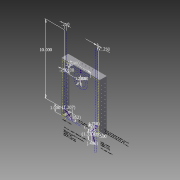
# Autodesk Inventor part: Bay Door Prototype Mk1
Saved by Autodesk Inventor 2015 (Build 190159000, 159)
## iProperties
Created: 2016-11-23
Part Number: Bay Door Prototype Mk1
Material: Generic
Document SubType Name: Modeling
Designer: Markus
Density: 1 g/cm^3
Appearance: Default
Author: Markus
Autodesk Inventor part; units mm, degrees
ref_plane "YZ Plane" through (0, 0, 0) normal (1, 0, 0) x (0, 1, 0)
ref_plane "XZ Plane" through (0, 0, 0) normal (0, 1, 0) x (-1, 0, 0)
ref_plane "XY Plane" through (0, 0, 0) normal (0, 0, 1) x (1, 0, 0)
sketch "Sketch1" plane through (0, 0, 0) normal (0, 0, 1) x (1, 0, 0)
  line L0 (0, 0) -> (142.24, 0)
  line L1 (142.24, 0) -> (142.24, 184.15)
  line L2 (142.24, 184.15) -> (0, 184.15)
  line L3 (0, 184.15) -> (0, 0)
  line L4 (4.3434, 179.8066) -> (137.8966, 179.8066)
  line L5 (137.8966, 179.8066) -> (137.8966, 4.3434)
  line L6 (137.8966, 4.3434) -> (4.3434, 4.3434)
  line L7 (4.3434, 4.3434) -> (4.3434, 179.8066)
  dimension "d0" = 184.15
  dimension "d1" = 142.24
  dimension "d2" = 4.3434
  constraints: 16 end point, 4 parallel, 2 perpendicular, 1 horizontal, 3 other
  measures "d0" distance of L2.end L0.start
  measures "d1" distance of L1.end L2.end
  measures "d2" distance between parallel lines of L2 L4
extrude "Extrusion1" add sketch "Sketch1" along normal blind 25.4
sketch "Sketch2" plane through (0, 0, 25.4) normal (0, 0, 1) x (1, 0, 0)
  line L0 (4.3434, 4.3434) -> (137.8966, 4.3434) projected
  line L1 (14.2875, 4.3434) -> (127.9525, 4.3434)
  line L2 (127.9525, 4.3434) -> (127.9525, 0)
  line L3 (127.9525, 0) -> (14.2875, 0)
  line L4 (14.2875, 0) -> (14.2875, 4.3434)
  line L5 (0, 184.15) -> (0, 0) projected
  line L6 (142.24, 0) -> (142.24, 184.15) projected
  dimension "d5" = 14.2875
  dimension "d6" = 14.2875
  constraints: 8 end point, 2 parallel, 1 horizontal, 1 horizontal alignment, 1 perpendicular, 1 point on line
  measures "d5" distance between parallel lines of L5 L4
  measures "d6" distance between parallel lines of L6 L2
extrude "Extrusion2" cut sketch "Sketch2" against normal up to surface (25.4 mm away)
sketch "Sketch3" plane through (0, 0, 25.4) normal (0, 0, 1) x (1, 0, 0)
  line L0 (10.6934, 279.4) -> (17.0434, 279.4) construction
  line L1 (17.0434, 279.4) -> (17.0434, 25.4) construction
  line L2 (17.0434, 25.4) -> (10.6934, 25.4) construction
  line L3 (10.6934, 25.4) -> (10.6934, 279.4) construction
  line L4 (125.1966, 279.4) -> (131.5466, 279.4) construction
  line L5 (131.5466, 279.4) -> (131.5466, 25.4) construction
  line L6 (131.5466, 25.4) -> (125.1966, 25.4) construction
  line L7 (125.1966, 25.4) -> (125.1966, 279.4) construction
  line L8 (14.2875, 4.3434) -> (71.12, 4.3434) construction
  line L9 (71.12, 4.3434) -> (71.12, 0) construction
  line L10 (71.12, 0) -> (14.2875, 0) construction
  line L11 (14.2875, 0) -> (14.2875, 4.3434) construction
  line L12 (4.3434, 179.8066) -> (137.8966, 179.8066) construction
  line L13 (4.3434, 4.3434) -> (4.3434, 179.8066) construction
  line L14 (0, 0) -> (14.2875, 0) construction
  line L15 (137.8966, 179.8066) -> (137.8966, 4.3434) construction
  line L16 (127.9525, 0) -> (123.6091, 0) construction
  line L17 (123.6091, 0) -> (123.6091, -56.8325) construction
  line L18 (123.6091, -56.8325) -> (127.9525, -56.8325) construction
  line L19 (127.9525, -56.8325) -> (127.9525, 0) construction
  line L20 (137.8966, 4.3434) -> (112.4966, 4.3434) construction
  arc A0 (111.9446, 7.4193) -> (112.4966, 4.3434) centre (112.4966, 5.9309) ccw construction
  line L21 (111.9446, 7.4193) -> (137.8966, 17.0434) construction
  line L22 (137.8966, 4.3434) -> (137.8966, 179.8066) construction
  line L23 (159.3941, 36.0216) -> (266.702, 36.0216) construction
  line L24 (266.702, 36.0216) -> (266.702, 6.9446) construction
  line L25 (266.702, 6.9446) -> (159.3941, 6.9446) construction
  line L26 (159.3941, 6.9446) -> (159.3941, 36.0216) construction
  circle A1 centre (13.8684, 28.575) radius 3.175 construction
  circle A2 centre (128.3716, 28.575) radius 3.175 construction
  line L27 (42.7037, 4.3434) -> (12.0379, 25.9808)
  line L28 (111.3731, 7.0524) -> (130.6186, 26.3319)
  line L29 (111.0091, 5.3763) -> (123.6091, -28.4162)
  line L30 (63.5032, 17.7448) -> (103.5407, 17.7448) construction
  line L31 (103.5407, 17.7448) -> (103.5407, 7.0443) construction
  line L32 (103.5407, 7.0443) -> (63.5032, 7.0443) construction
  line L33 (63.5032, 7.0443) -> (63.5032, 17.7448) construction
  line L34 (144.8974, -10.3874) -> (251.178, -10.3874) construction
  line L35 (251.178, -10.3874) -> (251.178, -62.6009) construction
  line L36 (251.178, -62.6009) -> (144.8974, -62.6009) construction
  line L37 (144.8974, -62.6009) -> (144.8974, -10.3874) construction
  arc A3 (111.3731, 7.0524) -> (111.0091, 5.3763) centre (112.4966, 5.9309) ccw
  line L38 (3.9911, -9.0202) -> (42.7037, -9.0202) construction
  line L39 (42.7037, -9.0202) -> (42.7037, -18.258) construction
  line L40 (42.7037, -18.258) -> (3.9911, -18.258) construction
  line L41 (3.9911, -18.258) -> (3.9911, -9.0202) construction
  line L42 (8.6414, -30.8758) -> (98.6277, -30.8758) construction
  line L43 (98.6277, -30.8758) -> (98.6277, -107.8338) construction
  line L44 (98.6277, -107.8338) -> (8.6414, -107.8338) construction
  line L45 (8.6414, -107.8338) -> (8.6414, -30.8758) construction
  circle A4 centre (71.12, 145.5166) radius 17.5641 construction
  line L46 (33.02, 179.8066) -> (109.22, 179.8066) construction
  line L47 (109.22, 179.8066) -> (109.22, 173.4566) construction
  line L48 (109.22, 173.4566) -> (33.02, 173.4566) construction
  line L49 (33.02, 173.4566) -> (33.02, 179.8066) construction
  circle A5 centre (71.12, 145.5166) radius 25.4 construction
  point P0 (71.12, 179.8066)
  point P1 (71.12, 179.8066)
  point P2 (71.12, 173.4566)
  point P3 (71.12, 179.8066)
  dimension "d9" = 6.35
  dimension "d10" = 6.35
  dimension "d11" = 25.4
  dimension "d12" = 254
  dimension "d13" = 6.35
  dimension "d14" = 25.4
  dimension "d15" = 3.175
  dimension "d16" = 12.7
  dimension "d34" = 30.6658
  dimension "d35" = 21.6374
  dimension "d36" = 19.2795
  dimension "d37" = 19.2456
  dimension "d38" = 33.7925
  dimension "d39" = 12.6
  dimension "d40" = 35.1282
  dimension "d41" = 6.35
  dimension "d42" = 50.8
  dimension "d43" = 27.94
  dimension "d44" = 76.2
  constraints: 50 end point, 10 parallel, 8 horizontal, 6 midpoint, 6 point on circle, 5 perpendicular, 4 centre point, 4 equal length, 4 tangent, 4 vertical, 4 vertical alignment, 3 coincident, 2 horizontal alignment, 2 point on line, 18 other
  measures "d9" distance between parallel lines of L1 L3
  measures "d10" distance between parallel lines of L13 L3
  measures "d11" distance between parallel lines of L14 L2
  measures "d12" distance of L2.end L0.start
  measures "d13" distance between parallel lines of L15 L5
  measures "d14" distance of L15.end L20.end
  measures "d15" diameter of A0
  measures "d16" distance from line of L20 L21.end
  measures "d34" horizontal distance of L27.start L27.end
  measures "d35" vertical distance of L27.start L27.end
  measures "d36" vertical distance of L28.start L28.end
  measures "d37" horizontal distance of L28.start L28.end
  measures "d38" vertical distance of L29.end L29.start
  measures "d39" horizontal distance of L29.start L29.end
  measures "d40" diameter of A4
  measures "d41" distance of L48.end L46.start
  measures "d42" diameter of A5
  measures "d43" distance from line of L48 A4.centre
  measures "d44" distance of L47.end L48.end
sketch "Sketch4" plane through (142.24, 0, 0) normal (1, 0, 0) x (0, 0, -1)
  line L0 (0, 4.3434) -> (-25.4, 4.3434) projected
  circle A0 centre (-19.05, 10.6934) radius 1.6129
  circle A1 centre (-6.35, 10.6934) radius 1.6129
  line L1 (-25.4, 17.0434) -> (-12.7, 4.3434) construction
  line L2 (0, 4.3434) -> (-25.4, 4.3434) construction
  line L3 (-12.7, 4.3434) -> (0, 17.0434) construction
  line L4 (0, 0) -> (0, 184.15) construction
  dimension "d17" = 3.2258
  constraints: 4 end point, 3 midpoint, 2 centre point, 1 equal radius, 1 perpendicular, 1 point on line
  measures "d17" diameter of A0
extrude "Extrusion3" cut sketch "Sketch4" against normal through all
pattern_linear "Rectangular Pattern1" count 13 spacing 12.7 along (0, 1, 0) of "Extrusion3"
sketch "Sketch6" plane through (0, 184.15, 0) normal (0, 1, 0) x (1, 0, 0)
  circle A0 centre (71.12, -6.35) radius 1.6129
  circle A1 centre (71.12, -19.05) radius 1.6129
  line L0 (142.24, 0) -> (0, 0) projected
  point P0 (71.12, 0)
  dimension "d23" = 3.2258
  dimension "d24" = 6.35
  dimension "d25" = 12.7
  constraints: 2 centre point, 2 vertical alignment, 1 equal radius, 1 midpoint
  measures "d23" diameter of A0
  measures "d24" distance from line of A0.centre L0
  measures "d25" distance of A0.centre A1.centre
extrude "Extrusion4" cut sketch "Sketch6" against normal up to surface (4.3434 mm away)
pattern_linear "Rectangular Pattern2" count 3 spacing 12.7 along (-1, 0, 0) count 3 spacing -12.7 along (-1, 0, 0) of "Extrusion4"
equation "\"d6\" = d5"
equation "\"d13\" = d10"
body "Solid1"
